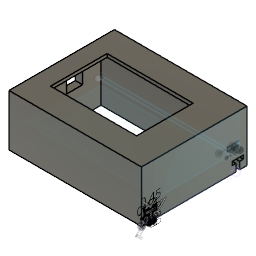
first_test_print_Ben_4 (Autodesk Fusion 360 design; units mm, degrees)
Autodesk Fusion 360 part; units mm, degrees
sketch "Sketch1" plane through (0, 0, 0) normal (0, 0, 1) x (1, 0, 0)
  line L0 (0, 0) -> (127, 0)
  line L1 (127, 0) -> (127, 68.58)
  line L2 (127, 68.58) -> (0, 68.58)
  line L3 (0, 68.58) -> (0, 0)
  line L4 (0, 0) -> (0, 34.29)
  line L5 (0, 34.29) -> (12.7, 34.29)
  line L6 (101.6, 0) -> (101.6, 63.5)
  line L7 (101.6, 63.5) -> (12.7, 63.5)
  line L8 (12.7, 63.5) -> (12.7, 0)
  line L9 (101.6, 5.08) -> (12.7, 5.08)
  dimension "d1" = 127
  dimension "d2" = 68.58
  dimension "d3" = 34.29
  dimension "d4" = 12.7
  dimension "d6" = 63.5
  constraint horizontal L0
  constraint vertical L1
  constraint horizontal L2
  constraint vertical L3
  constraint coincident L0.start L3.end
  constraint perpendicular L0 L4
  constraint perpendicular L3 L5
  constraint coincident L0 L6.start
  constraint perpendicular L0 L6
  constraint perpendicular L3 L7
  constraint coincident L0 L8.end
  constraint perpendicular L0 L8
  constraint coincident L6 L9.start
  constraint coincident L8 L9.end
  constraint perpendicular L8 L9
  measures "d1" distance of L0.start L0.end
  measures "d2" distance of L0.start L2.end
  measures "d3" distance of L0.start L4.end
  measures "d4" distance of L4.end L5.end
  measures "d6" distance of L6.start L6.end
extrude "Extrude1" add sketch "Sketch1" against normal blind 22.86 contours L0 L3 L4 L5 L8 | L0 L6 L8 L9 | L0 L1 L2 L3 L5 L6 L7 L8
sketch "Sketch2" plane through (0, 0, 0) normal (-1, 0, 0) x (0, -1, 0)
  line L0 (0, 0) -> (-68.58, 0)
  line L1 (-68.58, 0) -> (-68.58, -22.86)
  line L2 (-68.58, -22.86) -> (0, -22.86)
  line L3 (0, -22.86) -> (0, 0)
  line L4 (-68.58, -22.86) -> (-68.58, -20.32)
  line L5 (-27.94, -20.32) -> (-27.94, -6.35)
  line L6 (-27.94, -6.35) -> (-48.26, -6.35)
  line L7 (-48.26, -6.35) -> (-48.26, -20.32)
  line L8 (-48.26, -20.32) -> (-27.94, -20.32)
  dimension "d12" = 13.97
  constraint coincident L1.end L2.start
  constraint perpendicular L2 L4
  constraint perpendicular L5 L6
  constraint perpendicular L5 L8
  measures "d12" distance of L5.start L5.end
extrude "Extrude2" cut sketch "Sketch2" against normal blind 5.08 contours L5 L6 L7 L8
sketch "Sketch3" plane through (101.6, 0, 0) normal (-1, 0, 0) x (0, -1, 0)
  line L0 (-5.08, 0) -> (-63.5, 0)
  line L1 (-63.5, 0) -> (-63.5, -22.86)
  line L2 (-63.5, -22.86) -> (-5.08, -22.86)
  line L3 (-5.08, -22.86) -> (-5.08, 0)
  line L4 (-63.5, -22.86) -> (-63.5, -1.27)
  line L5 (-63.5, -1.27) -> (-5.08, -1.27)
  line L6 (-5.08, -22.86) -> (-5.08, -1.27)
  line L7 (-63.5, -22.86) -> (-5.08, -22.86)
  constraint coincident L1.end L2.start
  constraint coincident L1 L4.end
  constraint coincident L3 L5.end
  constraint perpendicular L3 L5
  constraint coincident L2.end L3.start
extrude "Extrude3" cut sketch "Sketch3" against normal blind 22.86 contours L1 L2 L3 L4 L5 L6 L7
sketch "Sketch4" plane through (12.7, 0, 0) normal (1, 0, 0) x (0, 1, 0)
  line L0 (63.5, 0) -> (5.08, 0)
  line L1 (5.08, 0) -> (5.08, -22.86)
  line L2 (5.08, -22.86) -> (63.5, -22.86)
  line L3 (63.5, -22.86) -> (63.5, 0)
  line L4 (5.08, -22.86) -> (5.08, -0.762)
  line L5 (5.08, -0.762) -> (63.5, -0.762)
  line L6 (63.5, -22.86) -> (63.5, -0.762)
  line L7 (63.5, -22.86) -> (5.08, -22.86)
  constraint coincident L1.end L2.start
  constraint coincident L1 L4.end
  constraint coincident L3 L5.end
  constraint perpendicular L3 L5
  constraint coincident L2.end L3.start
extrude "Extrude4" cut sketch "Sketch4" against normal blind 10.16 contours L1 L2 L3 L4 L5 L6 L7
sketch "Sketch5" plane through (0, 63.5, 0) normal (0, -1, 0) x (1, 0, 0)
  line L0 (101.6, 0) -> (12.7, 0)
  line L1 (12.7, 0) -> (12.7, -0.762)
  line L2 (12.7, -0.762) -> (2.54, -0.762)
  line L3 (2.54, -0.762) -> (2.54, -22.86)
  line L4 (2.54, -22.86) -> (124.46, -22.86)
  line L5 (124.46, -22.86) -> (124.46, -1.27)
  line L6 (124.46, -1.27) -> (101.6, -1.27)
  line L7 (101.6, -1.27) -> (101.6, 0)
  line L8 (2.54, -0.762) -> (124.46, -1.27)
  line L9 (124.46, -22.86) -> (2.54, -22.86)
  line L10 (2.54, -0.762) -> (2.54, -21.3653)
  constraint coincident L2.end L3.start
  constraint coincident L5.end L6.start
  constraint coincident L4.end L5.start
  constraint coincident L3.end L4.start
  constraint coincident L3 L10.end
extrude "Extrude5" cut sketch "Sketch5" against normal blind 3.81 contours L3 L4 L5 L6 L7 L8 L9 L10
sketch "Sketch6" plane through (0, 5.08, 0) normal (0, 1, 0) x (-1, 0, 0)
  line L0 (-12.7, 0) -> (-101.6, 0)
  line L1 (-101.6, 0) -> (-101.6, -1.27)
  line L2 (-101.6, -1.27) -> (-124.46, -1.27)
  line L3 (-124.46, -1.27) -> (-124.46, -22.86)
  line L4 (-124.46, -22.86) -> (-2.54, -22.86)
  line L5 (-2.54, -22.86) -> (-2.54, -0.762)
  line L6 (-2.54, -0.762) -> (-12.7, -0.762)
  line L7 (-12.7, -0.762) -> (-12.7, 0)
  line L8 (-124.46, -1.27) -> (-2.54, -0.762)
  line L9 (-2.54, -22.86) -> (-124.46, -22.86)
  line L10 (-124.46, -1.27) -> (-124.46, -22.86)
  constraint coincident L2.end L3.start
  constraint coincident L5.end L6.start
  constraint coincident L4.end L5.start
  constraint coincident L3.end L4.start
extrude "Extrude6" cut sketch "Sketch6" against normal blind 3.81 contours L1 L2 L3 L4 L5 L8 L9 L10
extrude "Extrude7" add 1 faces at (118.5333, 24.5533, 0) along direction (0, 0, 1) blind 2.54
extrude "Extrude8" add 1 faces at (0.8467, 27.94, -15.6633) along direction (0, 1, 0) blind 2.54
extrude "Extrude9" add 1 faces at (0.8467, 30.48, -15.6633) along direction (0, 1, 0) blind 1.27
extrude "Extrude10" add 1 faces at (118.5333, 24.5533, 2.54) along direction (0, 0, 1) blind 2.54
extrude "Extrude11" cut 1 faces at (116.84, 45.2967, -1.27) along direction (0, 0, 1) blind 2.54
extrude "Extrude12" cut 1 faces at (68.58, 2.54, -1.0372) along direction (0.004167, 0, 0.999991) blind 2.54
extrude "Extrude13" cut 1 faces at (35.56, 64.77, -0.8996) along direction (0.004167, 0, 0.999991) blind 2.54
extrude "Extrude14" cut 1 faces at (9.3133, 24.5533, -0.762) along direction (0, 0, 1) blind 2.54
extrude "Extrude15" add 1 faces at (42.3333, 0, -13.5467) along direction (0, -1, 0) blind 5.08
extrude "Extrude16" add 1 faces at (127, 44.0267, -13.5467) along direction (1, 0, 0) blind 5.08
extrude "Extrude17" add 1 faces at (88.0533, 68.58, -4.2333) along direction (0, 1, 0) blind 5.08
extrude "Extrude18" add 1 faces at (0, 7.1967, -8.0433) along direction (-1, 0, 0) blind 5.08
extrude "Extrude19" add 1 faces at (-2.54, 23.2833, -22.86) along direction (0, 0, -1) blind 7.62
sketch "Sketch7" plane through (0, 0, -30.48) normal (0, 0, -1) x (1, 0, 0)
  line L0 (132.08, 5.08) -> (-5.08, 5.08)
  line L1 (-5.08, 5.08) -> (-5.08, -73.66)
  line L2 (-5.08, -73.66) -> (132.08, -73.66)
  line L3 (132.08, -73.66) -> (132.08, 5.08)
  line L4 (2.54, -67.31) -> (2.54, -1.27)
  line L5 (2.54, -1.27) -> (124.46, -1.27)
  line L6 (124.46, -1.27) -> (124.46, -67.31)
  line L7 (124.46, -67.31) -> (2.54, -67.31)
extrude "Extrude20" add 1 faces at (40.64, 73.66, -18.6267) along direction (0, 1, 0) blind 7.62
sketch "Sketch8" plane through (0, 0, -30.48) normal (0, 0, -1) x (1, 0, 0)
  line L0 (132.08, 5.08) -> (-5.08, 5.08)
  line L1 (-5.08, 5.08) -> (-5.08, -81.28)
  line L2 (-5.08, -81.28) -> (132.08, -81.28)
  line L3 (132.08, -81.28) -> (132.08, 5.08)
  line L4 (2.54, -67.31) -> (2.54, -1.27)
  line L5 (2.54, -1.27) -> (124.46, -1.27)
  line L6 (124.46, -1.27) -> (124.46, -67.31)
  line L7 (124.46, -67.31) -> (2.54, -67.31)
  line L8 (124.46, -67.31) -> (124.46, -81.28)
  line L9 (132.08, -67.31) -> (132.08, -72.39)
  line L10 (132.08, -81.28) -> (132.08, -76.2)
  line L11 (-5.08, -76.2) -> (132.08, -76.2)
  line L12 (132.08, -72.39) -> (-5.08, -72.39)
  dimension "d51" = 5.08
  constraint coincident L6.end L7.start
  constraint coincident L2 L8.end
  constraint perpendicular L2 L8
  constraint coincident L3 L9.start
  constraint parallel L3 L9
  constraint coincident L2.end L3.start
  constraint coincident L3 L10.end
  constraint coincident L1 L11.start
  constraint perpendicular L3 L11
  constraint perpendicular L8 L12
  measures "d51" distance of L9.start L9.end
extrude "Extrude21" cut sketch "Sketch8" against normal blind 5.08 contours L1 L8 L11 L12
extrude "Extrude22" cut sketch "Sketch8" against normal blind 5.08 contours L3 L8 L11 L12
sketch "Sketch9" plane through (132.08, 0, 0) normal (1, 0, 0) x (0, 1, 0)
  line L0 (76.2, -25.4) -> (76.2, -30.48)
  line L1 (76.2, -30.48) -> (81.28, -30.48)
  line L2 (81.28, -30.48) -> (81.28, 5.08)
  line L3 (81.28, 5.08) -> (-5.08, 5.08)
  line L4 (-5.08, 5.08) -> (-5.08, -30.48)
  line L5 (-5.08, -30.48) -> (72.39, -30.48)
  line L6 (72.39, -30.48) -> (72.39, -25.4)
  line L7 (72.39, -25.4) -> (76.2, -25.4)
  line L8 (72.39, -25.4) -> (68.58, -25.4)
  line L9 (76.2, -25.4) -> (80.01, -25.4)
  line L10 (80.01, -25.4) -> (80.01, -21.59)
  line L11 (68.58, -25.4) -> (68.58, -21.59)
  line L12 (68.58, -21.59) -> (80.01, -21.59)
  dimension "d56" = 3.81
  dimension "d57" = 3.81
  dimension "d58" = 3.81
  constraint coincident L6.end L7.start
  constraint perpendicular L6 L8
  constraint coincident L0.start L7.end
  constraint perpendicular L0 L9
  constraint perpendicular L9 L10
  constraint perpendicular L8 L11
  measures "d56" distance of L6.end L8.end
  measures "d57" distance of L9.end L10.end
  measures "d58" distance of L8.end L11.end
extrude "Extrude23" add sketch "Sketch8" along normal blind 25.4 contours L0 L1 L3 L9 L12 | L1 L2 L8 L11 | L2 L3 L8 L10 L11
extrude "Extrude24" add 1 faces at (86.36, 74.93, -25.4) along direction (0, 0, -1) blind 25.4
extrude "Extrude25" add 1 faces at (86.36, 81.28, -15.24) along direction (0, 1, 0) blind 7.62
extrude "Extrude26" cut 1 faces at (86.36, 76.2, -52.4933) along direction (0, 1, 0) blind 7.62
extrude "Extrude27" add 1 faces at (86.36, 72.39, -54.1867) along direction (0, 1, 0) blind 7.62
extrude "Extrude28" cut 1 faces at (86.36, 80.01, -54.1867) along direction (0, -1, 0) blind 2.54
extrude "Extrude29" add 1 faces at (86.36, 83.82, -52.4933) along direction (0, -1, 0) blind 2.54
sketch "Sketch10" plane through (132.08, 0, 0) normal (1, 0, 0) x (0, 1, 0)
  line L0 (77.47, -55.88) -> (77.47, -50.8)
  line L1 (77.47, -50.8) -> (81.28, -50.8)
  line L2 (81.28, -50.8) -> (81.28, -55.88)
  line L3 (81.28, -55.88) -> (88.9, -55.88)
  line L4 (88.9, -55.88) -> (88.9, 5.08)
  line L5 (88.9, 5.08) -> (-5.08, 5.08)
  line L6 (-5.08, 5.08) -> (-5.08, -55.88)
  line L7 (-5.08, -55.88) -> (77.47, -55.88)
  line L8 (77.47, -50.8) -> (73.66, -50.8)
  line L9 (73.66, -50.8) -> (73.66, -46.99)
  line L10 (73.66, -46.99) -> (85.09, -46.99)
  line L11 (85.09, -46.99) -> (85.09, -50.8)
  line L12 (85.09, -50.8) -> (81.28, -50.8)
  dimension "d73" = 3.81
  dimension "d74" = 3.81
  dimension "d75" = 11.43
  constraint coincident L0.end L1.start
  constraint perpendicular L0 L8
  constraint perpendicular L8 L9
  constraint perpendicular L9 L10
  constraint perpendicular L10 L11
  constraint coincident L1.end L2.start
  constraint perpendicular L2 L12
  measures "d73" distance of L0.end L8.end
  measures "d74" distance of L8.end L9.end
  measures "d75" distance of L9.end L10.end
extrude "Extrude30" cut sketch "Sketch10" against normal blind 149.86 contours L1 L8 L9 L10 L11 L12
extrude "Extrude31" cut 1 faces at (86.36, 77.47, -46.99) along direction (0, 0, 1) blind 7.62
extrude "Extrude32" add 2 faces at (86.36, 83.82, -50.8) (40.64, 74.93, -50.8) along direction (0, 0, 1) blind 7.62
extrude "Extrude33" cut 2 faces at (43.18, 74.0833, -55.88) (86.36, 84.6667, -55.88) along direction (0, 0, 1) blind 7.62
extrude "Extrude34" cut 1 faces at (86.36, 77.47, -39.37) along direction (0, 0, 1) blind 2.54
extrude "Extrude35" add 2 faces at (86.36, 83.82, -43.18) (40.64, 74.93, -43.18) along direction (0, 0, 1) blind 2.54
sketch "Sketch11" plane through (0, 73.66, 0) normal (0, 1, 0) x (-1, 0, 0)
  line L0 (-132.08, -40.64) -> (5.08, -40.64)
  line L1 (5.08, -40.64) -> (5.08, -36.83)
  line L2 (5.08, -36.83) -> (-132.08, -36.83)
  line L3 (-132.08, -36.83) -> (-132.08, -40.64)
  line L4 (5.08, -40.64) -> (0, -40.64)
  line L5 (0, -36.83) -> (5.08, -36.83)
  line L6 (0, -40.64) -> (0, -36.83)
  constraint coincident L0.end L1.start
  constraint coincident L0 L4.end
  constraint coincident L2 L5.start
  constraint coincident L1.end L2.start
  constraint vertical L6
extrude "Extrude36" add sketch "Sketch11" along normal blind 11.43 contours L0 L1 L2 L4 L5 L6
sketch "Sketch12" plane through (0, 77.47, 0) normal (0, 1, 0) x (-1, 0, 0)
  line L0 (-132.08, -48.26) -> (5.08, -48.26)
  line L1 (5.08, -48.26) -> (5.08, -40.64)
  line L2 (5.08, -40.64) -> (0, -40.64)
  line L3 (0, -40.64) -> (-132.08, -40.64)
  line L4 (-132.08, -40.64) -> (-132.08, -48.26)
  line L5 (5.08, -40.64) -> (0, -40.64)
  line L6 (0, -40.64) -> (0, -48.26)
  line L7 (5.08, -48.26) -> (0, -48.26)
  line L8 (5.08, -48.26) -> (5.08, -40.64)
  dimension "d90" = 5.08
  constraint coincident L1.end L2.start
  constraint perpendicular L1 L5
  constraint coincident L0 L6.end
  constraint perpendicular L0 L6
  constraint coincident L0.end L1.start
  measures "d90" distance of L1.end L2.end
extrude "Extrude37" add sketch "Sketch12" along normal blind 3.81 contours L0 L1 L2 L5 L6 L7 L8
sketch "Sketch13" plane through (0, 0, -48.26) normal (0, 0, -1) x (1, 0, 0)
  line L0 (124.46, -1.27) -> (124.46, -67.31)
  line L1 (124.46, -67.31) -> (2.54, -67.31)
  line L2 (2.54, -67.31) -> (2.54, -1.27)
  line L3 (2.54, -1.27) -> (124.46, -1.27)
  line L4 (-5.08, 5.08) -> (-5.08, -88.9)
  line L5 (-5.08, -88.9) -> (132.08, -88.9)
  line L6 (132.08, -88.9) -> (132.08, -81.28)
  line L7 (132.08, -81.28) -> (0, -81.28)
  line L8 (0, -81.28) -> (0, -77.47)
  line L9 (0, -77.47) -> (132.08, -77.47)
  line L10 (132.08, -77.47) -> (132.08, 5.08)
  line L11 (132.08, 5.08) -> (-5.08, 5.08)
extrude "Extrude38" add 1 faces at (86.36, -5.08, -12.7) along direction (0, -1, 0) blind 15.24
sketch "Sketch14" plane through (0, 0, -48.26) normal (0, 0, -1) x (1, 0, 0)
  line L0 (124.46, -1.27) -> (124.46, 8.89)
  line L1 (132.08, -77.47) -> (132.08, 20.32)
  line L2 (124.46, 8.89) -> (132.08, 8.89)
  line L3 (132.08, 20.32) -> (132.08, 12.7)
  point P0 (124.46, -1.27)
  dimension "d95" = 10.16
  constraint coincident P0 L0.start
  constraint coincident L1 L2.end
  constraint perpendicular L0 L2
  constraint coincident L1.end L3.start
  constraint coincident L1 L3.end
  measures "d95" distance of P0 L0.end
sketch "Sketch15" plane through (132.08, 0, 0) normal (1, 0, 0) x (0, 1, 0)
  line L0 (73.66, -40.64) -> (73.66, -36.83)
  line L1 (73.66, -36.83) -> (85.09, -36.83)
  line L2 (85.09, -36.83) -> (85.09, -40.64)
  line L3 (85.09, -40.64) -> (81.28, -40.64)
  line L4 (81.28, -40.64) -> (81.28, -48.26)
  line L5 (81.28, -48.26) -> (88.9, -48.26)
  line L6 (88.9, -48.26) -> (88.9, 5.08)
  line L7 (88.9, 5.08) -> (-20.32, 5.08)
  line L8 (-20.32, 5.08) -> (-20.32, -48.26)
  line L9 (-20.32, -48.26) -> (77.47, -48.26)
  line L10 (77.47, -48.26) -> (77.47, -40.64)
  line L11 (77.47, -40.64) -> (73.66, -40.64)
  line L12 (-12.7, -48.26) -> (-12.7, -40.64)
  line L13 (-8.89, -48.26) -> (-8.89, -40.64)
  line L14 (-12.7, -40.64) -> (-16.51, -40.64)
  line L15 (-16.51, -40.64) -> (-16.51, -36.83)
  line L16 (-16.51, -36.83) -> (-5.08, -36.83)
  line L17 (-5.08, -36.83) -> (-5.08, -40.64)
  line L18 (-5.08, -40.64) -> (-8.89, -40.64)
  point P0 (-12.7, -48.26)
  point P1 (-8.89, -48.26)
  dimension "d96" = 7.62
  dimension "d97" = 7.62
  dimension "d98" = 3.81
  dimension "d99" = 3.81
  dimension "d100" = 11.43
  constraint coincident P0 L12.start
  constraint perpendicular L9 L12
  constraint coincident P1 L13.start
  constraint perpendicular L9 L13
  constraint perpendicular L12 L14
  constraint perpendicular L14 L15
  constraint perpendicular L12 L16
  constraint perpendicular L16 L17
  constraint perpendicular L17 L18
  measures "d96" distance of P0 L12.end
  measures "d97" distance of P1 L13.end
  measures "d98" distance of L12.end L14.end
  measures "d99" distance of L14.end L15.end
  measures "d100" distance of L15.end L16.end
